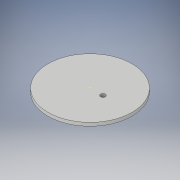
# Autodesk Inventor part: WireSpoolSide
Saved by Autodesk Inventor 2018 (Build 220112000, 112)
## iProperties
Created: 2017-11-17
Part Number: WireSpoolSide
Material: Generic
Document SubType Name: Modeling
Designer: ball
Density: 1 g/cm^3
Appearance: Default
Author: ball
Autodesk Inventor part; units mm, degrees
ref_plane "YZ Plane" through (0, 0, 0) normal (1, 0, 0) x (0, 1, 0)
ref_plane "XZ Plane" through (0, 0, 0) normal (0, 1, 0) x (-1, 0, 0)
ref_plane "XY Plane" through (0, 0, 0) normal (0, 0, 1) x (1, 0, 0)
sketch "Sketch1" plane through (0, 0, 0) normal (0, 1, 0) x (-1, 0, 0)
  circle A0 centre (0, 0) radius 31.75
  circle A1 centre (9.779, 0) radius 1.778
  circle A2 centre (0, 9.779) radius 1.778
  circle A3 centre (-9.779, 0) radius 1.778
  circle A4 centre (0, -9.779) radius 1.778
  dimension "d0" = 63.5
  dimension "d3" = 3.556
  dimension "d6" = 360
  constraints: 5 centre point, 2 coincident, 9 other
  measures "d0" diameter of A0
  measures "d3" diameter of A1
extrude "Extrusion1" add sketch "Sketch1" along normal blind 2.54 contours A0 | A1 | A2 | A3 | A4
sketch "Sketch2" plane through (0, 2.54, 0) normal (0, 1, 0) x (1, 0, 0)
  point P0 (0, 0)
sketch "Sketch3" plane through (0, 2.54, 0) normal (0, 1, 0) x (1, 0, 0)
  circle A0 centre (9.779, 0) radius 1.778
  point P0 (0, 0)
  dimension "d8" = 3.556
  constraints: 1 centre point, 1 coincident
  measures "d8" diameter of A0
hole "Hole1" at (9.779, 2.54, 0) direction (0, -1, 0) diameter 3.556 end through all
body "Solid1"
